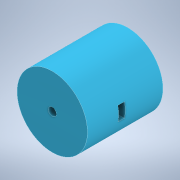
# Autodesk Inventor part: DestinationSpoolHolder
Saved by Autodesk Inventor 2021 (Build 250183000, 183)
## iProperties
Created: 2021-03-09
Part Number: DestinationSpoolHolder
Material: Generic
Document SubType Name: Modeling
Designer: elmar
Density: 1 g/cm^3
Appearance: Turquoise
Author: elmar
Autodesk Inventor part; units mm, degrees
ref_plane "YZ Plane" through (0, 0, 0) normal (1, 0, 0) x (0, 1, 0)
ref_plane "XZ Plane" through (0, 0, 0) normal (0, 1, 0) x (-1, 0, 0)
ref_plane "XY Plane" through (0, 0, 0) normal (0, 0, 1) x (1, 0, 0)
sketch "Sketch2" plane through (0, 0, 0) normal (0, 0, 1) x (1, 0, 0)
  circle A0 centre (0, 0) radius 14
  dimension "d1" = 28
  constraints: 1 centre point, 1 coincident
  measures "d1" diameter of A0
extrude "Extrusion1" add sketch "Sketch2" along normal mid plane 30
sketch "Sketch3" plane through (0, 0, 15) normal (0, 0, 1) x (1, 0, 0)
  point P0 (0, 0)
hole "Hole1" at (0, 0, 15) direction (0, 0, -1) diameter 3.2 depth 5 clearance for "Flat Head Machine Screw" size "M3" standard "Ansi Metric M Profile"
sketch "Sketch4" plane through (0, 0, 10) normal (0, 0, 1) x (1, 0, 0)
  circle A0 centre (0, 0) radius 1.6 projected
  line L0 (-1.5877, 2.75) -> (1.5877, 2.75)
  line L1 (1.5877, 2.75) -> (3.1754, 0)
  line L2 (3.1754, 0) -> (1.5877, -2.75)
  line L3 (1.5877, -2.75) -> (-1.5877, -2.75)
  line L4 (-1.5877, -2.75) -> (-3.1754, 0)
  line L5 (-3.1754, 0) -> (-1.5877, 2.75)
  dimension "d11" = 5.5
  constraints: 12 end point, 1 coincident, 1 horizontal, 13 other
  measures "d11" distance between parallel lines of L3 L0
extrude "Extrusion2" cut sketch "Sketch4" against normal up to surface (10 mm away) contours A0 | L0 L1 L2 L3 L4 L5
sketch "Sketch5" plane through (0, 0, -15) normal (0, 0, -1) x (-1, 0, 0)
  circle A0 centre (0, 0) radius 2.5
  line L0 (-1.5, 2) -> (1.5, 2)
  dimension "d41" = 5
  dimension "d42" = 4.5
  constraints: 2 end point, 2 point on circle, 1 centre point, 1 coincident, 1 horizontal
  measures "d41" diameter of A0
extrude "Extrusion3" cut sketch "Sketch5" against normal up to surface (15 mm away) contours A0 L0 picked at (0.1119, 0.5076)
sketch "Sketch8" plane through (0, 0, 0) normal (1, 0, 0) x (0, 1, 0)
  line L0 (2.85, 0) -> (-2.85, 0)
  line L1 (-2.85, 0) -> (-2.85, 2.6)
  line L2 (-2.85, 2.6) -> (2.85, 2.6)
  line L3 (2.85, 2.6) -> (2.85, 0)
  point P0 (0, 0)
  dimension "d48" = 2.6
  dimension "d49" = 5.7
  constraints: 8 end point, 2 parallel, 1 horizontal, 1 midpoint, 1 perpendicular
  measures "d48" distance of L2.end L0.start
  measures "d49" distance of L1.end L2.end
extrude "Extrusion4" cut sketch "Sketch8" along normal through all both and the other way through all
equation "\"d30\" = 55deg"
equation "\"Sketch6_Pitch\" = 1.25"
body "Solid1"
